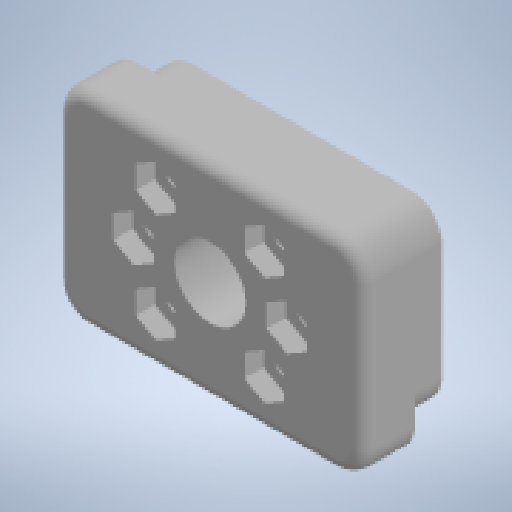
# Autodesk Inventor part: 2x3_Spacer_Rear
Saved by Autodesk Inventor 2023 (Build 270158000, 158)
## iProperties
Created: 2022-05-03
Part Number: 2x3_Spacer_Rear
Material: Generic
Document SubType Name: Modeling
Designer: plebbb
Density: 1 g/cm^3
Appearance: Default
Mass: 109.593 g
Surface Area: 204.871 cm^2
Volume: 109.593 cm^3
Author: plebbb
Autodesk Inventor part; units mm, degrees
ref_plane "YZ Plane" through (0, 0, 0) normal (1, 0, 0) x (0, 1, 0)
ref_plane "XZ Plane" through (0, 0, 0) normal (0, 1, 0) x (-1, 0, 0)
sketch "Sketch1" plane through (0, 0, 0) normal (0, 0, 1) x (1, 0, 0)
  line L0 (7.62, 0) -> (61.595, 0)
  line L1 (69.215, 7.62) -> (69.215, 36.195)
  line L2 (61.595, 43.815) -> (7.62, 43.815)
  line L3 (0, 36.195) -> (0, 7.62)
  arc A0 (7.62, 43.815) -> (0, 36.195) centre (7.62, 36.195) ccw
  arc A1 (0, 7.62) -> (7.62, 0) centre (7.62, 7.62) ccw
  arc A2 (61.595, 0) -> (69.215, 7.62) centre (61.595, 7.62) ccw
  arc A3 (69.215, 36.195) -> (61.595, 43.815) centre (61.595, 36.195) ccw
  point P0 (0, 0)
  point P1 (69.215, 43.815)
  point P2 (69.215, 0)
  point P3 (0, 43.815)
  dimension "d0" = 69.215
  dimension "d1" = 43.815
  dimension "d2" = 7.62
  constraints: 8 end point, 8 point on circle, 8 point on line, 8 tangent, 4 centre point, 3 equal radius, 2 parallel, 1 horizontal, 1 perpendicular
  measures "d0" distance of point (69.215, 43.815) point (0, 43.815)
  measures "d1" distance of point (69.215, 0) point (69.215, 43.815)
  measures "d2" radius of A0
extrude "Extrusion1" add sketch "Sketch1" along normal blind 9
sketch "Sketch2" plane through (0, 0, 9) normal (0, 0, 1) x (1, 0, 0)
  line L0 (4.1275, -3.4925) -> (65.0875, -3.4925)
  line L1 (72.7075, 4.1275) -> (72.7075, 39.6875)
  line L2 (65.0875, 47.3075) -> (4.1275, 47.3075)
  line L3 (-3.4925, 39.6875) -> (-3.4925, 4.1275)
  arc A0 (4.1275, 47.3075) -> (-3.4925, 39.6875) centre (4.1275, 39.6875) ccw
  arc A1 (-3.4925, 4.1275) -> (4.1275, -3.4925) centre (4.1275, 4.1275) ccw
  arc A2 (65.0875, -3.4925) -> (72.7075, 4.1275) centre (65.0875, 4.1275) ccw
  arc A3 (72.7075, 39.6875) -> (65.0875, 47.3075) centre (65.0875, 39.6875) ccw
  line L4 (61.595, 43.815) -> (7.62, 43.815) construction
  line L5 (0, 36.195) -> (0, 7.62) construction
  point P0 (0, 0)
  point P1 (72.7075, 47.3075)
  point P2 (72.7075, -3.4925)
  point P3 (-3.4925, 47.3075)
  point P4 (34.6075, 47.3075)
  point P5 (34.6075, 43.815)
  point P6 (-3.4925, 21.9075)
  point P7 (0, 21.9075)
  dimension "d5" = 76.2
  dimension "d6" = 50.8
  dimension "d7" = 7.62
  constraints: 8 end point, 8 point on circle, 8 tangent, 6 point on line, 4 centre point, 4 midpoint, 3 equal radius, 2 parallel, 1 horizontal, 1 horizontal alignment, 1 perpendicular, 1 vertical alignment
  measures "d5" distance of point (72.707, 47.307) point (-3.492, 47.308)
  measures "d6" distance of point (72.707, -3.493) point (72.707, 47.307)
  measures "d7" radius of A0
extrude "Extrusion2" add sketch "Sketch2" along normal blind 12.7
fillet "Fillet1" radius 3.175 8 edges at (-1.2607, 45.0757, 21.7) (-3.4925, 21.9075, 21.7) (-1.2607, -1.2607, 21.7) (34.6075, -3.4925, 21.7) (70.4757, -1.2607, 21.7) (72.7075, 21.9075, 21.7) (70.4757, 45.0757, 21.7) (34.6075, 47.3075, 21.7)
sketch "Sketch3" plane through (0, 0, 21.7) normal (0, 0, 1) x (1, 0, 0)
  line L0 (65.0875, 47.3075) -> (4.1275, 47.3075) construction
  line L1 (65.0875, 47.3075) -> (4.1275, 47.3075) construction
  line L2 (-3.4925, 39.6875) -> (-3.4925, 4.1275) construction
  line L3 (-3.4925, 39.6875) -> (-3.4925, 4.1275) construction
  circle A0 centre (34.6075, 21.9075) radius 8.75
  circle A1 centre (34.6075, 21.9075) radius 19 construction
  circle A2 centre (21.1725, 35.3425) radius 2.25
  circle A3 centre (48.0425, 35.3425) radius 2.25
  circle A4 centre (15.6075, 21.9075) radius 2.25
  circle A5 centre (53.6075, 21.9075) radius 2.25
  circle A6 centre (21.1725, 8.4725) radius 2.25
  circle A7 centre (48.0425, 8.4725) radius 2.25
  line L4 (21.1725, 35.3425) -> (34.6075, 21.9075) construction
  line L5 (34.6075, 21.9075) -> (15.6075, 21.9075) construction
  point P0 (0, 0)
  point P1 (34.6075, 47.3075)
  point P2 (-3.4925, 21.9075)
  point P3 (-3.4925, 21.9075)
  dimension "d11" = 17.5
  dimension "d14" = 4.5
  dimension "d15" = 38
  dimension "d16" = 45
  constraints: 8 centre point, 6 point on circle, 5 equal radius, 5 horizontal alignment, 4 end point, 3 midpoint, 3 vertical alignment, 1 coincident
  measures "d11" diameter of A0
  measures "d14" diameter of A2
  measures "d15" diameter of A1
  measures "d16" angle of L5 L4
extrude "Extrusion3" cut sketch "Sketch3" against normal up to surface (21.7 mm away)
chamfer "Chamfer1" distance 1.27 angle 45 6 edges at (45.7925, 35.3425, 0) (18.9225, 35.3425, 0) (13.3575, 21.9075, 0) (51.3575, 21.9075, 0) (45.7925, 8.4725, 0) (18.9225, 8.4725, 0)
sketch "Sketch4" plane through (7.62, 0, 0) normal (0, -1, 0) x (1, 0, 0)
  point P0 (-7.62, 0)
ref_plane "Work Plane1" through (-0.635, 46.99, -50.8) normal (0, 1, 0) x (0, 0, 1)
sketch "Sketch7" plane through (0, 0, 21.7) normal (0, 0, 1) x (1, 0, 0)
  line L0 (21.1725, 2.7532) -> (16.2195, 5.6129)
  line L1 (16.2195, 5.6129) -> (16.2195, 11.3321)
  line L2 (16.2195, 11.3321) -> (21.1725, 14.1917)
  line L3 (21.1725, 14.1917) -> (26.1255, 11.3321)
  line L4 (26.1255, 11.3321) -> (26.1255, 5.6129)
  line L5 (26.1255, 5.6129) -> (21.1725, 2.7532)
  circle A0 centre (48.0425, 35.3425) radius 2.25 construction
  circle A1 centre (53.6075, 21.9075) radius 2.25 construction
  circle A2 centre (48.0425, 8.4725) radius 2.25 construction
  circle A3 centre (21.1725, 8.4725) radius 2.25 construction
  circle A4 centre (15.6075, 21.9075) radius 2.25 construction
  circle A5 centre (21.1725, 35.3425) radius 2.25 construction
  line L6 (53.6075, 16.1883) -> (48.6545, 19.0479)
  line L7 (48.6545, 19.0479) -> (48.6545, 24.7671)
  line L8 (48.6545, 24.7671) -> (53.6075, 27.6267)
  line L9 (53.6075, 27.6267) -> (58.5605, 24.7671)
  line L10 (58.5605, 24.7671) -> (58.5605, 19.0479)
  line L11 (58.5605, 19.0479) -> (53.6075, 16.1883)
  line L12 (48.0425, 29.6233) -> (43.0895, 32.4829)
  line L13 (43.0895, 32.4829) -> (43.0895, 38.2021)
  line L14 (43.0895, 38.2021) -> (48.0425, 41.0618)
  line L15 (48.0425, 41.0618) -> (52.9955, 38.2021)
  line L16 (52.9955, 38.2021) -> (52.9955, 32.4829)
  line L17 (52.9955, 32.4829) -> (48.0425, 29.6233)
  line L18 (15.6075, 16.1883) -> (10.6545, 19.0479)
  line L19 (10.6545, 19.0479) -> (10.6545, 24.7671)
  line L20 (10.6545, 24.7671) -> (15.6075, 27.6267)
  line L21 (15.6075, 27.6267) -> (20.5605, 24.7671)
  line L22 (20.5605, 24.7671) -> (20.5605, 19.0479)
  line L23 (20.5605, 19.0479) -> (15.6075, 16.1883)
  line L24 (21.1725, 29.6233) -> (16.2195, 32.4829)
  line L25 (16.2195, 32.4829) -> (16.2195, 38.2021)
  line L26 (16.2195, 38.2021) -> (21.1725, 41.0618)
  line L27 (21.1725, 41.0618) -> (26.1255, 38.2021)
  line L28 (26.1255, 38.2021) -> (26.1255, 32.4829)
  line L29 (26.1255, 32.4829) -> (21.1725, 29.6233)
  line L30 (48.0425, 2.7532) -> (43.0895, 5.6129)
  line L31 (43.0895, 5.6129) -> (43.0895, 11.3321)
  line L32 (43.0895, 11.3321) -> (48.0425, 14.1917)
  line L33 (48.0425, 14.1917) -> (52.9955, 11.3321)
  line L34 (52.9955, 11.3321) -> (52.9955, 5.6129)
  line L35 (52.9955, 5.6129) -> (48.0425, 2.7532)
  point P0 (0, 0)
  dimension "d26" = 9.906
  constraints: 72 end point, 6 coincident, 6 vertical, 5 parallel, 78 other
  measures "d26" distance between parallel lines of L1 L4
extrude "Extrusion6" cut sketch "Sketch7" against normal blind 4.7625
body "Solid1"
